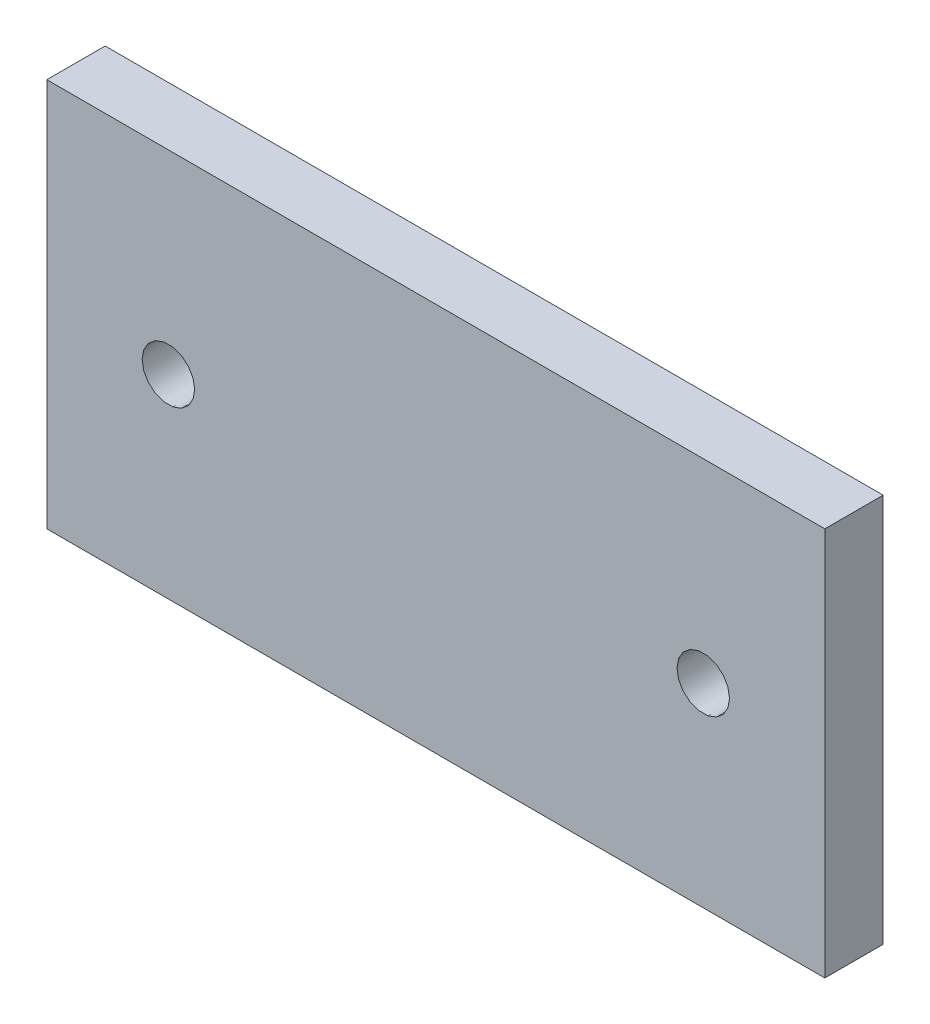
# Autodesk Inventor part: Part4
Saved by Autodesk Inventor 2016 SP1 (Build 200210100, 210)
## iProperties
Created: 2016-03-17
Part Number: Part4
Material: Generic
Document SubType Name: Modeling
Designer: Mohamed A.
Density: 1 g/cm^3
Appearance: Default
Author: Mohamed A.
Autodesk Inventor part; units mm, degrees
ref_plane "YZ Plane" through (0, 0, 0) normal (1, 0, 0) x (0, 1, 0)
ref_plane "XZ Plane" through (0, 0, 0) normal (0, 1, 0) x (-1, 0, 0)
ref_plane "XY Plane" through (0, 0, 0) normal (0, 0, 1) x (1, 0, 0)
sketch "Sketch1" plane through (0, 0, 0) normal (0, 0, 1) x (1, 0, 0)
  line L0 (-20, 10) -> (20, 10)
  line L1 (20, 10) -> (20, -10)
  line L2 (20, -10) -> (-20, -10)
  line L3 (-20, -10) -> (-20, 10)
  line L4 (-20, 10) -> (20, -10) construction
  line L5 (20, 10) -> (-20, -10) construction
  line L6 (7.5, 25) -> (-7.5, 25) construction
  line L7 (-7.5, 25) -> (-7.5, -25) construction
  line L8 (-7.5, -25) -> (7.5, -25) construction
  line L9 (7.5, -25) -> (7.5, 25) construction
  line L10 (-28, 0) -> (28, 0) construction
  circle A0 centre (13.75, 0) radius 1.35
  circle A1 centre (-13.75, 0) radius 1.35
  point P0 (0, 0)
  dimension "d0" = 40
  dimension "d1" = 20
  dimension "d2" = 2.7
  dimension "d3" = 2.7
  dimension "d4" = 12.5
  dimension "d5" = 6.25
  dimension "d6" = 6.25
  constraints: 12 end point, 2 centre point, 2 midpoint, 2 parallel, 2 point on line, 1 horizontal, 1 perpendicular
  measures "d0" distance of L1.end L2.end
  measures "d1" distance of L0.end L1.end
  measures "d2" diameter of A0
  measures "d3" diameter of A1
  measures "d4" distance between parallel lines of L9 L1
  measures "d5" distance from line of L9 A0.centre
  measures "d6" distance from line of L7 A1.centre
extrude "Extrusion1" add sketch "Sketch1" along normal blind 3
equation "\"d5\" = 0.5 * d4"
equation "\"d6\" = d5"
body "Solid1"
